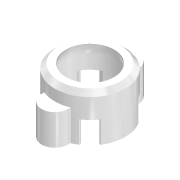
# Autodesk Inventor part: Ш.04.Корпус
Saved by Autodesk Inventor 2021.3 (Build 253353010, 353A)
## iProperties
Created: 2021-07-07
Part Number: Ш.04.Корпус
Material: ABS Plastic
Document SubType Name: Modeling
Designer: Михальчик
Density: 1.06 g/cm^3
Appearance: Smooth - White
Author: Михальчик
Autodesk Inventor part; units mm, degrees
ref_plane "YZ Plane" through (0, 0, 0) normal (1, 0, 0) x (0, 1, 0)
ref_plane "XZ Plane" through (0, 0, 0) normal (0, 1, 0) x (-1, 0, 0)
ref_plane "XY Plane" through (0, 0, 0) normal (0, 0, 1) x (1, 0, 0)
sketch "Sketch1" plane through (0, 0, 0) normal (0, 1, 0) x (-1, 0, 0)
  circle A0 centre (0, 0) radius 8
  circle A1 centre (0, -8) radius 3
  circle A2 centre (0, 8) radius 3
  line L0 (0, 8) -> (0, -8) construction
  circle A3 centre (0, 8) radius 1.1
  circle A4 centre (0, -8) radius 1.1
  circle A5 centre (0, 0) radius 6
  circle A6 centre (4.242641, 4.242641) radius 2
  circle A7 centre (0, 0) radius 4 construction
  circle A8 centre (-4.242641, -4.242641) radius 2
  line L1 (-4.242641, -4.242641) -> (4.242641, 4.242641) construction
  circle A9 centre (4.242641, 4.242641) radius 2.5 construction
  line L2 (6.717514, 4.596194) -> (4.596194, 6.717514) construction
  line L3 (-4.117395, -6.238715) -> (-6.238715, -4.117395)
  line L4 (-4.117395, -6.238715) -> (-4.40662, -6.676953)
  line L5 (-6.238715, -4.117395) -> (-6.676953, -4.40662)
  circle A10 centre (4.242641, -4.242641) radius 2
  line L6 (6.238715, -4.117395) -> (6.676953, -4.40662)
  line L7 (4.117395, -6.238715) -> (4.40662, -6.676953)
  circle A11 centre (4.242641, 4.242641) radius 2
  line L8 (4.117395, 6.238715) -> (4.40662, 6.676953)
  line L9 (6.238715, 4.117395) -> (6.676953, 4.40662)
  circle A12 centre (-4.242641, 4.242641) radius 2
  line L10 (-6.238715, 4.117395) -> (-6.676953, 4.40662)
  line L11 (-4.117395, 6.238715) -> (-4.40662, 6.676953)
  point P0 (-2.946794, 7.4375)
  point P1 (-2.946794, -7.4375)
  point P2 (2.946794, -7.4375)
  point P3 (2.946794, 7.4375)
  point P4 (1.911111, 5.6875)
  point P5 (1.911111, -5.6875)
  point P6 (-1.911111, -5.6875)
  point P7 (-1.911111, 5.6875)
  point P8 (-2.612505, 5.401372)
  point P9 (-5.401372, 2.612505)
  point P10 (2.612505, 5.401372)
  point P11 (5.401372, 2.612505)
  point P12 (2.612505, -5.401372)
  point P13 (5.401372, -2.612505)
  point P14 (-2.612505, -5.401372)
  point P15 (-5.401372, -2.612505)
  dimension "d0" = 16
  dimension "d1" = 6
  dimension "d2" = 6
  dimension "d3" = 2.2
  dimension "d4" = 2.2
  dimension "d5" = 12
  dimension "d10" = 45
  dimension "d11" = 4
  dimension "d12" = 3
  dimension "d13" = 3
  dimension "d16" = 360
  constraints: 24 end point, 14 point on circle, 13 centre point, 7 coincident, 5 tangent, 2 line through centre, 2 midpoint, 2 perpendicular, 1 vertical, 33 other
  measures "d0" diameter of A0
  measures "d1" diameter of A1
  measures "d2" diameter of A2
  measures "d3" diameter of A3
  measures "d4" diameter of A4
  measures "d5" diameter of A5
  measures "d10" angle of L0 L1
  measures "d11" diameter of A6
  measures "d12" distance of L2.start L2.end
  measures "d13" distance of L3.start L3.end
extrude "Extrusion1" add sketch "Sketch1" along normal blind 7 contours A0 L6 A10 A5 A6 L9 | L9 A6 A0 | A0 A10 L6 | A6 L8 A0 | A6 A5 | A0 L7 A10 | A10 A5 | L8 A6 A5 A2 A0 | A0 A1 A5 A10 L7 | A2 A5 A0 A3 | A0 A3 A2 | A1 A0 A4 | A0 A4 A1 A5 | A3 A0 | A0 A3 | A4 A0 | A0 A4 | A5 A12 L11 A0 A2 | A0 L4 A8 A5 A1 | A5 A12 | L11 A12 A0 | A0 A8 L4 | A8 L3 A5 | A5 A8 L5 A0 L10 A12 | A12 L10 A0 | A0 L5 A8 | A8 L3 picked at (4.69644, 4.69644) picked at (4.69644, -4.69644) picked at (-4.69644, 4.69644)
extrude "Extrusion3" add sketch "Sketch1" along normal blind 10.5 contours A0 L6 A10 A5 A6 L9 | L9 A6 A0 | A0 A10 L6 | A6 L8 A0 | A6 A5 | A0 L7 A10 | A10 A5 | L8 A6 A5 A2 A0 | A0 A1 A5 A10 L7 | A2 A5 A0 A3 | A0 A4 A1 A5 | A3 A0 | A0 A4 | A5 A12 L11 A0 A2 | A0 L4 A8 A5 A1 | A5 A12 | L11 A12 A0 | A0 A8 L4 | A8 L3 A5 | A5 A8 L5 A0 L10 A12 | A12 L10 A0 | A0 L5 A8 | A8 L3 picked at (4.69644, 4.69644) picked at (4.69644, -4.69644) picked at (0.04227, 7.630168) picked at (0.04227, -7.630168) picked at (-4.69644, 4.69644)
extrude "Extrusion2" cut sketch "Sketch1" along normal blind 5 contours L9 A6 A0 | A0 A10 L6 | A6 L8 A0 | A6 A5 | A0 L7 A10 | A10 A5 | A3 A0 | A0 A3 | A4 A0 | A0 A4 | A5 A12 | L11 A12 A0 | A0 A8 L4 | A8 L3 A5 | A12 L10 A0 | A0 L5 A8 | A8 L3 picked at (4.69644, 4.69644) picked at (4.69644, -4.69644) picked at (-4.69644, 4.69644)
fillet "Fillet1" radius 0.2 27 edges at (-6.677, 2.5, -4.4066) (-6.2387, 2.5, -4.1174) (-5.4014, 2.5, -2.6125) (-4.4066, 2.5, -6.677) (-4.1174, 2.5, -6.2387) (-2.6125, 2.5, -5.4014) (-5.4014, 2.5, 2.6125) (-6.2387, 2.5, 4.1174) (-6.677, 2.5, 4.4066) (-4.4066, 2.5, 6.677) (-4.1174, 2.5, 6.2387) (-2.6125, 2.5, 5.4014) (5.4014, 2.5, 2.6125) (6.2387, 2.5, -4.1174) (6.677, 2.5, -4.4066) (4.1174, 2.5, -6.2387) (4.4066, 2.5, -6.677) (4.1174, 2.5, 6.2387) (4.4066, 2.5, 6.677) (6.2387, 2.5, 4.1174) (6.677, 2.5, 4.4066) (2.9468, 3.5, 7.4375) (-2.9468, 3.5, 7.4375) (-2.9468, 3.5, -7.4375) (2.9468, 3.5, -7.4375) (5.4014, 2.5, -2.6125) (2.6125, 2.5, -5.4014)
chamfer "Chamfer1" distance 1 angle 45 1 edges at (8, 10.5, 0)
sketch "Sketch2" plane through (0, 0, 0) normal (1, 0, 0) x (0, 1, 0)
  circle A0 centre (8, 0) radius 6
  line L0 (10.5, 6) -> (0, 6)
  line L1 (10.5, 6) -> (10.5, 5.454356)
  line L2 (0, 0) -> (8, 0)
  point P0 (8, 6)
  dimension "d24" = 12
  dimension "d25" = 8
  constraints: 4 end point, 1 parallel, 1 perpendicular, 3 other
  measures "d25" distance of L2.start L2.end
revolve "Revolution1" add sketch "Sketch2" angle 360 about axis through (0, 0, 0) along (0, 1, 0) contours A0 L0 L1
body "Solid1"
